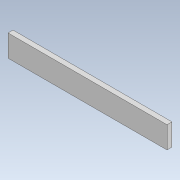
# Autodesk Inventor part: Part5
Saved by Autodesk Inventor 2020 (Build 240168000, 168)
## iProperties
Created: 2021-01-23
Part Number: Part5
Material: Generic
Document SubType Name: Modeling
Designer: DELL
Density: 1 g/cm^3
Appearance: Default
Author: DELL
Autodesk Inventor part; units mm, degrees
ref_plane "YZ Plane" through (0, 0, 0) normal (1, 0, 0) x (0, 1, 0)
ref_plane "XZ Plane" through (0, 0, 0) normal (0, 1, 0) x (-1, 0, 0)
ref_plane "XY Plane" through (0, 0, 0) normal (0, 0, 1) x (1, 0, 0)
sketch "Sketch1" plane through (0, 0, 0) normal (1, 0, 0) x (0, 1, 0)
  line L0 (11, -2.5) -> (-11, -2.5)
  line L1 (-11, -2.5) -> (-11, 2.5)
  line L2 (-11, 2.5) -> (11, 2.5)
  line L3 (11, 2.5) -> (11, -2.5)
  line L4 (11, -2.5) -> (-11, 2.5) construction
  line L5 (-11, -2.5) -> (11, 2.5) construction
  point P0 (0, 0)
  dimension "d0" = 5
  dimension "d1" = 22
  constraints: 12 end point, 2 midpoint, 2 parallel, 1 horizontal, 1 perpendicular
  measures "d0" distance of L0.end L1.end
  measures "d1" distance of L0.start L0.end
extrude "Extrusion1" add sketch "Sketch1" along normal mid plane 160
sketch "Sketch2" plane through (0, 0, 0) normal (0, 0, 1) x (1, 0, 0)
  line L0 (80, 11) -> (-80, 11) projected
  line L1 (0, 11) -> (98, 11)
  line L2 (98, 11) -> (110, -1)
  line L3 (110, -1) -> (110, -11)
  line L4 (110, -11) -> (0, -11)
  line L5 (-80, -11) -> (80, -11) projected
  line L6 (0, 11) -> (0, -11) construction
  line L7 (-80, 11) -> (80, 11) construction
  line L8 (-80, -11) -> (-80, 11) construction
  line L9 (-80, -11) -> (80, -11) construction
  line L10 (80, 11) -> (80, -11) construction
  line L11 (-80, 11) -> (80, 11) construction
  line L12 (-80, -11) -> (-80, 11) construction
  line L13 (-80, -11) -> (80, -11) construction
  line L14 (0, 11) -> (-98, 11)
  line L15 (-98, 11) -> (-110, -1)
  line L16 (-110, -1) -> (-110, -11)
  line L17 (-110, -11) -> (0, -11)
  point P0 (-80, 11)
  dimension "d8" = 45
  dimension "d9" = 110
  dimension "d10" = 10
  constraints: 18 end point, 3 symmetric about line, 2 collinear, 2 midpoint, 2 perpendicular
  measures "d8" angle of L4 L2
  measures "d9" distance between parallel lines of L6 L3
  measures "d10" distance of L2.end L3.end
body "Solid1"
